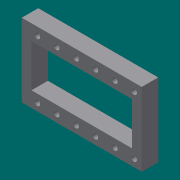
# Autodesk Inventor part: 知能ロボコンタミヤギアモータ用マウントスペーサ
Saved by Autodesk Inventor 2013 (Build 170138000, 138)
## iProperties
Created: 2014-09-06
Part Number: 知能ロボコンタミヤギアモータ用マウントスペーサ
Material: 一般
Document SubType Name: Modeling
Designer: horumo136
Density: 1 g/cm^3
Author: horumo136
Autodesk Inventor part; units mm, degrees
ref_plane "YZ Plane" through (0, 0, 0) normal (1, 0, 0) x (0, 1, 0)
ref_plane "XZ Plane" through (0, 0, 0) normal (0, 1, 0) x (-1, 0, 0)
ref_plane "XY Plane" through (0, 0, 0) normal (0, 0, 1) x (1, 0, 0)
sketch "スケッチ1" plane through (0, 0, 0) normal (0, 1, 0) x (-1, 0, 0)
  circle A0 centre (4, 34) radius 1.5
  circle A1 centre (44, 34) radius 1.5
  circle A2 centre (24, 34) radius 1.5
  circle A3 centre (44, 4) radius 1.5
  circle A4 centre (24, 4) radius 1.5
  circle A5 centre (4, 4) radius 1.5
  circle A6 centre (14, 4) radius 1.5
  circle A7 centre (34, 4) radius 1.5
  circle A8 centre (54, 4) radius 1.5
  circle A9 centre (34, 34) radius 1.5
  circle A10 centre (54, 34) radius 1.5
  circle A11 centre (14, 34) radius 1.5
  line L0 (0, 0) -> (62, 0)
  line L1 (62, 0) -> (62, 38)
  line L2 (62, 38) -> (0, 38)
  line L3 (0, 38) -> (0, 0)
  constraints: 12 centre point, 8 end point
extrude "押し出し1" add sketch "スケッチ1" along normal blind 8.5
sketch "スケッチ2" plane through (0, 0, 0) normal (0, -1, 0) x (1, 0, 0)
  line L0 (0, 0) -> (-62, 0) projected
  line L1 (0, 38) -> (0, 0) projected
  line L2 (-62, 38) -> (0, 38) projected
  line L3 (-62, 0) -> (-62, 38) projected
  line L4 (-57, 30) -> (-5, 30)
  line L5 (-5, 30) -> (-5, 8)
  line L6 (-5, 8) -> (-57, 8)
  line L7 (-57, 8) -> (-57, 30)
  dimension "d2" = 5
  dimension "d3" = 5
  dimension "d4" = 8
  dimension "d5" = 8
  constraints: 8 end point, 2 parallel, 1 horizontal, 1 perpendicular
  measures "d2" distance between parallel lines of L7 L3
  measures "d3" distance between parallel lines of L1 L5
  measures "d4" distance between parallel lines of L2 L4
  measures "d5" distance between parallel lines of L0 L6
extrude "押し出し2" cut sketch "スケッチ2" against normal through all contours L4 L5 L6 L7
